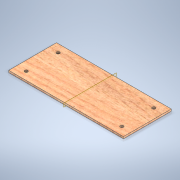
# Autodesk Inventor part: Side Plane
Saved by Autodesk Inventor 2020.2 (Build 242310000, 310)
## iProperties
Created: 2020-03-05
Part Number: Side Plane
Material: Wood (Birch)
Document SubType Name: Modeling
Designer: sdekr
Density: 0.55 g/cm^3
Appearance: Birch - Natural Polished
Author: sdekr
Autodesk Inventor part; units mm, degrees
ref_plane "YZ Plane" through (0, 0, 0) normal (1, 0, 0) x (0, 1, 0)
ref_plane "XZ Plane" through (0, 0, 0) normal (0, 1, 0) x (-1, 0, 0)
ref_plane "XY Plane" through (0, 0, 0) normal (0, 0, 1) x (1, 0, 0)
sketch "Sketch1" plane through (0, 0, 0) normal (0, 1, 0) x (-1, 0, 0)
  line L0 (-90, 37.5) -> (90, 37.5)
  line L1 (90, 37.5) -> (90, -37.5)
  line L2 (90, -37.5) -> (-90, -37.5)
  line L3 (-90, -37.5) -> (-90, 37.5)
  line L4 (-90, 37.5) -> (90, -37.5) construction
  line L5 (90, 37.5) -> (-90, -37.5) construction
  point P0 (0, 0)
  dimension "d0" = 180
  dimension "d1" = 75
  constraints: 12 end point, 2 midpoint, 2 parallel, 1 horizontal, 1 perpendicular
  measures "d0" distance of L1.end L2.end
  measures "d1" distance of L0.end L1.end
extrude "Extrusion1" add sketch "Sketch1" along normal blind 3
sketch "Sketch2" plane through (0, 0, 0) normal (0, -1, 0) x (1, 0, 0)
  circle A0 centre (75, 25) radius 2.4
  circle A1 centre (75, -25) radius 2.4
  circle A2 centre (97.5, 25) radius 2.7 projected
  circle A3 centre (97.5, -25) radius 2.7 projected
  line L0 (90, 37.5) -> (90, -37.5) projected
  point P0 (0, 0)
  dimension "d4" = 4.8
  dimension "d5" = 15
  constraints: 2 centre point, 2 horizontal alignment, 1 equal radius, 1 vertical alignment
  measures "d4" diameter of A0
  measures "d5" distance from line of L0 A1.centre
ref_plane "Work Plane1" through (0, 0, 37.5) normal (1, 0, 0) x (0, 0, -1)
extrude "Extrusion2" cut sketch "Sketch2" against normal through all contours A0 | A1
mirror "Mirror1" about plane through (0, 0, 37.5) normal (1, 0, 0) of "Extrusion2"
body "Solid1"
